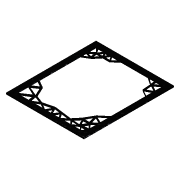
# Autodesk Inventor part: FrontCover
Saved by Autodesk Inventor 2014 (Build 180170000, 170)
## iProperties
Created: 2014-08-10
Part Number: FrontCover
Material: Generic
Document SubType Name: Modeling
Designer: Peele
Density: 1 g/cm^3
Appearance: Black
Author: Peele
Autodesk Inventor part; units mm, degrees
ref_plane "YZ Plane" through (0, 0, 0) normal (1, 0, 0) x (0, 1, 0)
ref_plane "XZ Plane" through (0, 0, 0) normal (0, 1, 0) x (-1, 0, 0)
ref_plane "XY Plane" through (0, 0, 0) normal (0, 0, 1) x (1, 0, 0)
sketch "Sketch1" plane through (0, 0, 0) normal (0, 0, 1) x (1, 0, 0)
  line L0 (-112.5, -130) -> (112.5, -130)
  line L1 (112.5, -130) -> (112.5, 130)
  line L2 (112.5, 130) -> (-112.5, 130)
  line L3 (-112.5, 130) -> (-112.5, -130)
  line L4 (-112.5, -130) -> (112.5, 130) construction
  line L5 (112.5, -130) -> (-112.5, 130) construction
  point P0 (0, 0)
  dimension "d0" = 225
  dimension "d1" = 260
  constraints: 12 end point, 2 midpoint, 2 parallel, 1 horizontal, 1 perpendicular
  measures "d0" distance of L1.end L2.end
  measures "d1" distance of L2.end L0.start
extrude "Extrusion1" add sketch "Sketch1" along normal blind 4
sketch "Sketch2" plane through (0, 0, 4) normal (0, 0, 1) x (1, 0, 0)
  line L0 (112.5, -130) -> (112.5, 130) projected
  line L1 (112.5, 130) -> (-112.5, 130) projected
  line L2 (-97.5, -115) -> (97.5, -115) construction
  line L3 (97.5, -115) -> (97.5, 115) construction
  line L4 (97.5, 115) -> (-97.5, 115) construction
  line L5 (-97.5, 115) -> (-97.5, -115) construction
  line L6 (-97.5, -115) -> (97.5, 115) construction
  line L7 (97.5, -115) -> (-97.5, 115) construction
  line L8 (-97.5, 69.6214) -> (-97.5, -49.3315)
  line L9 (-97.5, -49.3315) -> (-74.2083, -62.6108)
  line L10 (-74.2083, -62.6108) -> (-60.4842, -92.6336)
  line L11 (-60.4842, -92.6336) -> (-36.2885, -101.8837)
  line L12 (-36.2885, -101.8837) -> (-5.3522, -94.1478)
  line L13 (-5.3522, -94.1478) -> (44.4287, -100.7131)
  line L14 (44.4287, -100.7131) -> (59.884, -82.4839)
  line L15 (59.884, -82.4839) -> (74.8264, -56.275)
  line L16 (74.8264, -56.275) -> (97.5, -37.0517)
  line L17 (97.5, -37.0517) -> (97.5, 63.3607)
  line L18 (97.5, 63.3607) -> (76.5718, 75.2925)
  line L19 (76.5718, 75.2925) -> (74.8264, 99.5832)
  line L20 (74.8264, 99.5832) -> (51.4726, 115)
  line L21 (51.4726, 115) -> (-24.6752, 115)
  line L22 (-24.6752, 115) -> (-43.3511, 99.1661)
  line L23 (-43.3511, 99.1661) -> (-62.4247, 99.1661)
  line L24 (-62.4247, 99.1661) -> (-76.8543, 82.1466)
  line L25 (-76.8543, 82.1466) -> (-97.5, 69.6214)
  line L26 (-97.5, -53.3316) -> (-77.8137, -64.4134)
  line L27 (-77.8137, -64.4134) -> (-97.5, -77.7402)
  line L28 (-97.5, -53.3316) -> (-97.5, -77.7402)
  line L29 (-75.9334, -67.1347) -> (-64.1189, -92.9802)
  line L30 (-64.1189, -92.9802) -> (-94.8838, -79.9633)
  line L31 (-94.8838, -79.9633) -> (-75.9334, -67.1347)
  line L32 (-97.5, -80.8061) -> (-67.2206, -94.5022)
  line L33 (-67.2206, -94.5022) -> (-97.5, -115)
  line L34 (-97.5, -80.8061) -> (-97.5, -115)
  line L35 (-61.8122, -95.0679) -> (-39.5333, -103.5852)
  line L36 (-39.5333, -103.5852) -> (-58.3487, -115)
  line L37 (-61.8122, -95.0679) -> (-58.3487, -115)
  line L38 (-93.2759, -115) -> (-62.2536, -115)
  line L39 (-62.2536, -115) -> (-65.212, -97.9743)
  line L40 (-65.212, -97.9743) -> (-93.2759, -115)
  line L41 (-33.6147, -104.2979) -> (-5.4112, -97.2453)
  line L42 (-5.4112, -97.2453) -> (-14.8228, -115.0117)
  line L43 (-14.8228, -115.0117) -> (-33.6147, -104.2979)
  line L44 (-37.0725, -105.2517) -> (-53.1409, -115)
  line L45 (-37.0725, -105.2517) -> (-18.6705, -115)
  line L46 (-18.6705, -115) -> (-53.1409, -115)
  line L47 (-4.0054, -97.0003) -> (15.5053, -99.5735)
  line L48 (15.5053, -99.5735) -> (5.3216, -115)
  line L49 (-4.0054, -97.0003) -> (5.3216, -115)
  line L50 (17.9527, -99.6172) -> (42.9141, -102.9092)
  line L51 (42.9141, -102.9092) -> (28.6532, -115)
  line L52 (18.2678, -99.6587) -> (28.6532, -115)
  line L53 (-5.1316, -101.2632) -> (-12.4086, -115)
  line L54 (-5.1316, -101.2632) -> (1.9865, -115)
  line L55 (-12.4086, -115) -> (1.9865, -115)
  line L56 (16.6142, -102.1788) -> (8.1504, -115)
  line L57 (16.6142, -102.1788) -> (24.3926, -115)
  line L58 (8.1504, -115) -> (24.3926, -115)
  line L59 (97.5, -39.6957) -> (76.6353, -57.3854)
  line L60 (76.6353, -57.3854) -> (97.5, -67.4979)
  line L61 (97.5, -39.6957) -> (97.5, -67.4979)
  line L62 (74.9846, -60.0737) -> (62.9914, -82.7135)
  line L63 (62.9914, -82.7135) -> (80.6459, -82.7135)
  line L64 (80.6459, -82.7135) -> (74.9846, -60.0737)
  line L65 (77.9221, -60.8557) -> (97.5, -70.3445)
  line L66 (77.9221, -60.8557) -> (83.3044, -82.3799)
  line L67 (83.3044, -82.3799) -> (97.5, -70.3445)
  line L68 (97.5, -74.8014) -> (86.1632, -84.413)
  line L69 (86.1632, -84.413) -> (97.5, -97.7846)
  line L70 (97.5, -74.8014) -> (97.5, -97.7846)
  line L71 (62.9789, -85.2945) -> (48.2128, -100.9654)
  line L72 (48.2128, -100.9654) -> (72.1328, -102.96)
  line L73 (72.1328, -102.96) -> (62.9789, -85.2945)
  line L74 (46.1245, -102.797) -> (33.4701, -115)
  line L75 (46.1245, -102.797) -> (57.8922, -115)
  line L76 (33.4701, -115) -> (57.8922, -115)
  line L77 (52.352, -102.8432) -> (72.8995, -104.5565)
  line L78 (72.8995, -104.5565) -> (60.5816, -115)
  line L79 (52.352, -102.8432) -> (60.5816, -115)
  line L80 (66.7406, -86.293) -> (74.4295, -101.1313)
  line L81 (74.4295, -101.1313) -> (82.9052, -85.1315)
  line L82 (82.9052, -85.1315) -> (66.7406, -86.293)
  line L83 (85.2228, -89.2985) -> (77.4115, -101.1313)
  line L84 (77.4115, -101.1313) -> (96.3376, -99.7714)
  line L85 (96.3376, -99.7714) -> (85.2228, -89.2985)
  line L86 (75.6266, -104.8036) -> (63.6001, -115)
  line L87 (86.4479, -115) -> (75.6266, -104.8036)
  line L88 (79.974, -104.8036) -> (97.5, -104.8036)
  line L89 (79.974, -104.8036) -> (88.6188, -115)
  line L90 (97.5, -104.8036) -> (88.6188, -115)
  line L91 (93.0594, -115) -> (97.5, -108.2732)
  line L92 (93.0594, -115) -> (97.5, -115)
  line L93 (97.5, -108.2732) -> (97.5, -115)
  line L94 (86.4479, -115) -> (63.6001, -115)
  line L95 (97.1167, 64.7922) -> (78.1163, 75.6249)
  line L96 (78.1163, 75.6249) -> (97.5, 85.4001)
  line L97 (97.1167, 64.7922) -> (97.5, 85.4001)
  line L98 (97.5, 88.3594) -> (78.8792, 78.2226)
  line L99 (78.8792, 78.2226) -> (77.3852, 99.015)
  line L100 (77.3852, 99.015) -> (97.5, 88.3594)
  line L101 (79.6739, 100.7493) -> (97.5, 91.3061)
  line L102 (97.5, 115) -> (79.6739, 100.7493)
  line L103 (97.5, 91.3061) -> (97.5, 115)
  line L104 (75.6266, 115) -> (76.5718, 101.846)
  line L105 (76.5718, 101.846) -> (93.026, 115)
  line L106 (75.6266, 115) -> (93.026, 115)
  line L107 (72.8995, 115) -> (73.8447, 101.846)
  line L108 (73.8447, 101.846) -> (56.4668, 115)
  line L109 (56.4668, 115) -> (72.8995, 115)
  line L110 (-28.7528, 115) -> (-42.3934, 101.846)
  line L111 (-42.3934, 101.846) -> (-51.2981, 115)
  line L112 (-28.7528, 115) -> (-51.2981, 115)
  line L113 (-54.4466, 115) -> (-45.5419, 101.846)
  line L114 (-45.5419, 101.846) -> (-61.7739, 102.1479)
  line L115 (-61.7739, 102.1479) -> (-54.4466, 115)
  line L116 (-80.1773, 81.9074) -> (-97.5, 71.3981)
  line L117 (-97.5, 71.3981) -> (-97.5, 86.1839)
  line L118 (-97.5, 86.1839) -> (-80.1773, 81.9074)
  line L119 (-66.5334, 99.1665) -> (-78.5907, 83.2375)
  line L120 (-78.5907, 83.2375) -> (-80.7926, 99.4317)
  line L121 (-80.7926, 99.4317) -> (-66.5334, 99.1665)
  line L122 (-83.0801, 99.1661) -> (-81.0249, 84.0513)
  line L123 (-81.0249, 84.0513) -> (-95.8931, 88.3029)
  line L124 (-95.8931, 88.3029) -> (-83.0801, 99.1661)
  line L125 (-97.5, 90.0921) -> (-84.285, 101.2961)
  line L126 (-84.285, 101.2961) -> (-97.5, 115)
  line L127 (-97.5, 90.0921) -> (-97.5, 115)
  line L128 (-90.8925, 115) -> (-81.6155, 101.2961)
  line L129 (-81.6155, 101.2961) -> (-72.569, 115)
  line L130 (-90.8925, 115) -> (-72.569, 115)
  line L131 (-71.5186, 113.6071) -> (-78.5374, 101.2961)
  line L132 (-78.5374, 101.2961) -> (-65.891, 101.2961)
  line L133 (-65.891, 101.2961) -> (-71.5186, 113.6071)
  line L134 (-69.026, 113.6071) -> (-58.1103, 113.6071)
  line L135 (-58.1103, 113.6071) -> (-63.9698, 102.546)
  line L136 (-63.9698, 102.546) -> (-69.026, 113.6071)
  point P0 (0, 0)
  dimension "d4" = 15
  dimension "d5" = 15
  constraints: 262 end point, 52 parallel, 32 perpendicular, 4 collinear, 4 horizontal, 3 vertical, 2 midpoint, 1 point on line, 61 other
extrude "Extrusion2" cut sketch "Sketch2" against normal blind 4
body "Solid1"
